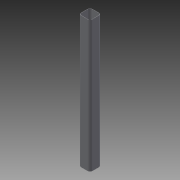
# Autodesk Inventor part: SmallCFTube
Saved by Autodesk Inventor 2015 (Build 190159000, 159)
## iProperties
Created: 2018-05-03
Part Number: SmallCFTube
Material: Generic
Document SubType Name: Modeling
Designer: HP USER
Density: 1 g/cm^3
Appearance: Default
Author: HP USER
Autodesk Inventor part; units mm, degrees
ref_plane "YZ Plane" through (0, 0, 0) normal (1, 0, 0) x (0, 1, 0)
ref_plane "XZ Plane" through (0, 0, 0) normal (0, 1, 0) x (-1, 0, 0)
sketch "Sketch1" plane through (0, 0, 0) normal (0, 0, 1) x (1, 0, 0)
  line L0 (3, 3) -> (3, -3) projected
  line L1 (6.35, -6.35) -> (3, -3) projected
  line L2 (6.35, -6.35) -> (6.35, -7.652) projected
  line L3 (-6.35, -7.652) -> (6.35, -7.652) projected
  line L4 (-6.35, -7.652) -> (-6.35, -6.35) projected
  line L5 (-3, -3) -> (-6.35, -6.35) projected
  line L6 (-3, -3) -> (-3, 3) projected
  line L7 (-6.35, 6.35) -> (-3, 3) projected
  line L8 (-6.35, 6.35) -> (-6.35, 7.652) projected
  line L9 (6.35, 7.652) -> (-6.35, 7.652) projected
  line L10 (6.35, 7.652) -> (6.35, 6.35) projected
  line L11 (3, 3) -> (6.35, 6.35) projected
  arc A0 (-6.0001, 10.0001) -> (-10.0001, 6.0001) centre (-6.0001, 6.0001) ccw projected
  line L12 (-10.0001, 6.0001) -> (-10.0001, -6.0001) projected
  arc A1 (-10.0001, -6.0001) -> (-6.0001, -10.0001) centre (-6.0001, -6.0001) ccw projected
  line L13 (-6.0001, -10.0001) -> (6.0001, -10.0001) projected
  arc A2 (6.0001, -10.0001) -> (10.0001, -6.0001) centre (6.0001, -6.0001) ccw projected
  line L14 (10.0001, -6.0001) -> (10.0001, 6.0001) projected
  arc A3 (10.0001, 6.0001) -> (6.0001, 10.0001) centre (6.0001, 6.0001) ccw projected
  line L15 (6.0001, 10.0001) -> (-6.0001, 10.0001) projected
  line L16 (-10.5001, -6.0001) -> (-10.5001, 6.0001)
  arc A4 (-6.0001, 10.5001) -> (-10.5001, 6.0001) centre (-6.0001, 6.0001) ccw
  line L17 (-6.0001, 10.5001) -> (6.0001, 10.5001)
  arc A5 (10.5001, 6.0001) -> (6.0001, 10.5001) centre (6.0001, 6.0001) ccw
  line L18 (10.5001, 6.0001) -> (10.5001, -6.0001)
  arc A6 (6.0001, -10.5001) -> (10.5001, -6.0001) centre (6.0001, -6.0001) ccw
  line L19 (6.0001, -10.5001) -> (-6.0001, -10.5001)
  arc A7 (-10.5001, -6.0001) -> (-6.0001, -10.5001) centre (-6.0001, -6.0001) ccw
  point P0 (0, 0)
  dimension "d0" = 0.5
  constraints: 8 end point, 8 point on circle, 4 centre point, 7 other
  measures "d0" distance between parallel lines of L12 L16
ref_plane "Work Plane1" through (-10.9987, -11, -15) normal (0, 0, 1) x (1, 0, 0)
extrude "Extrusion1" add sketch "Sketch1" against normal up to surface (15 mm away) contours L16 A4 L17 A5 L18 A6 L19 A7
sketch "Sketch2" plane through (0, 0, 0) normal (0, 0, 1) x (1, 0, 0)
  line L0 (-10.0001, -6.0001) -> (-10.0001, 6.0001) projected
  arc A0 (-6.0001, 10.0001) -> (-10.0001, 6.0001) centre (-6.0001, 6.0001) ccw projected
  line L1 (-6.0001, 10.0001) -> (6.0001, 10.0001) projected
  arc A1 (10.0001, 6.0001) -> (6.0001, 10.0001) centre (6.0001, 6.0001) ccw projected
  line L2 (10.0001, 6.0001) -> (10.0001, -6.0001) projected
  arc A2 (6.0001, -10.0001) -> (10.0001, -6.0001) centre (6.0001, -6.0001) ccw projected
  line L3 (6.0001, -10.0001) -> (-6.0001, -10.0001) projected
  arc A3 (-10.0001, -6.0001) -> (-6.0001, -10.0001) centre (-6.0001, -6.0001) ccw projected
  line L4 (-10.5001, -6.0001) -> (-10.5001, 6.0001) projected
  arc A4 (-10.5001, -6.0001) -> (-6.0001, -10.5001) centre (-6.0001, -6.0001) ccw projected
  line L5 (6.0001, -10.5001) -> (-6.0001, -10.5001) projected
  arc A5 (6.0001, -10.5001) -> (10.5001, -6.0001) centre (6.0001, -6.0001) ccw projected
  line L6 (10.5001, 6.0001) -> (10.5001, -6.0001) projected
  arc A6 (10.5001, 6.0001) -> (6.0001, 10.5001) centre (6.0001, 6.0001) ccw projected
  line L7 (-6.0001, 10.5001) -> (6.0001, 10.5001) projected
  arc A7 (-6.0001, 10.5001) -> (-10.5001, 6.0001) centre (-6.0001, 6.0001) ccw projected
  point P0 (0, 0)
extrude "Extrusion2" add sketch "Sketch2" along normal blind 230
body "Solid1"
